Autodesk Inventor part; units mm, degrees
(part 2 of 2)
  circle A256 centre (0, -145) radius 6.25 projected
  circle A257 centre (102.5305, -102.5305) radius 6.25 projected
  circle A258 centre (145, 0) radius 6.25 projected
  circle A259 centre (102.5305, 102.5305) radius 6.25 projected
  circle A260 centre (0, 0) radius 126 projected
  circle A261 centre (0, 0) radius 375
  dimension "d60" = 750
  constraints: 1 centre point, 1 coincident
  measures "d60" diameter of A261
extrude "Extrusion4" cut sketch "Sketch5" against normal through all contours A260 | A261
equation "\"d0\" = da_da"
equation "\"d1\" = da_b"
equation "\"d49\" = Вал_ось_диаметр_НОС"
equation "\"d3\" = da_d"
equation "\"d16\" = da_aw"
equation "\"d43\" = da_aw"
equation "\"d46\" = da_aw"
equation "\"BendRadius\" = Thickness"
equation "\"BendReliefWidth\" = Thickness"
equation "\"BendReliefDepth\" = 0.5 * Thickness"
equation "\"CornerReliefSize\" = 4 * Thickness"
equation "\"MinimumRemnant\" = 2 * Thickness"
equation "\"TransitionRadius\" = BendRadius"
equation "\"JacobiRadiusSize\" = BendRadius"
equation "\"GapSize\" = Thickness"
equation "\"da_da\" = 812.91152"
equation "\"da_b\" = 24"
equation "\"Вал_ось_диаметр_НОС\" = 250"
equation "\"da_d\" = 787.89816"
equation "\"da_aw\" = 494"
equation "\"Thickness\" = 24"
body "Solid1"
body "Srf1"
